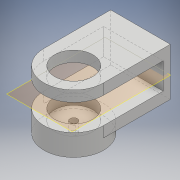
# Autodesk Inventor part: baseRotor1
Saved by Autodesk Inventor 2017 (Build 210142000, 142)
## iProperties
Created: 2017-08-06
Part Number: baseRotor1
Material: Generic
Document SubType Name: Sheet Metal
Designer: Bardo91
Density: 1 g/cm^3
Sheet Metal Rule: Default_mm
Appearance: Default
Author: Bardo91
Autodesk Inventor part; units mm, degrees
ref_plane "YZ Plane" through (0, 0, 0) normal (1, 0, 0) x (0, 1, 0)
ref_plane "XZ Plane" through (0, 0, 0) normal (0, 1, 0) x (-1, 0, 0)
ref_plane "XY Plane" through (0, 0, 0) normal (0, 0, 1) x (1, 0, 0)
sketch "Sketch1" plane through (0, 0, 0) normal (0, 0, 1) x (1, 0, 0)
  circle A0 centre (0, 0) radius 16
  circle A1 centre (0, 0) radius 25
  line L0 (-25, 0) -> (-25, 50)
  line L1 (-25, 50) -> (25, 50)
  line L2 (25, 50) -> (25, 0)
  dimension "d0" = 32
  dimension "d1" = 50
  dimension "d2" = 50
  dimension "d3" = 50
  constraints: 6 end point, 2 centre point, 2 coincident, 2 perpendicular, 2 point on circle, 1 vertical
  measures "d0" diameter of A0
  measures "d1" diameter of A1
  measures "d2" distance of L0.start L0.end
  measures "d3" distance of L0.end L1.end
extrude "Extrusion1" add sketch "Sketch1" along normal blind 9
ref_plane "Work Plane1" through (0, 0, -11) normal (0, 0, 1) x (1, 0, 0)
mirror "Mirror1" about plane through (0, 0, -11) normal (0, 0, 1) of "Extrusion1"
sketch "Sketch2" plane through (0, 0, -31) normal (0, 0, -1) x (-1, 0, 0)
  circle A0 centre (0, 0) radius 16 projected
  circle A1 centre (0, 0) radius 25
  dimension "d11" = 50
  constraints: 1 centre point, 1 coincident
  measures "d11" diameter of A1
extrude "Extrusion2" add sketch "Sketch2" along normal blind 9 contours A0 | A1
sketch "Sketch3" plane through (0, 0, -31) normal (0, 0, 1) x (1, 0, 0)
  circle A0 centre (0, 0) radius 3.1
  dimension "d14" = 6.2
  constraints: 1 centre point, 1 coincident
  measures "d14" diameter of A0
extrude "Extrusion3" cut sketch "Sketch3" against normal blind 1
sketch "Sketch4" plane through (0, 0, -32) normal (0, 0, 1) x (1, 0, 0)
  circle A0 centre (0, 0) radius 3.1
  line L0 (0, 0) -> (0, -1.5)
  line L1 (0, -1.5) -> (-2.7129, -1.5)
  line L2 (0, -1.5) -> (2.7129, -1.5)
  dimension "d17" = 6.2
  dimension "d18" = 1.5
  constraints: 6 end point, 2 horizontal, 2 point on circle, 1 centre point, 1 coincident, 1 vertical
  measures "d17" diameter of A0
  measures "d18" distance of L0.start L0.end
extrude "Extrusion4" cut sketch "Sketch4" against normal through all contours A0 L2 L1 picked at (-0.0193, 1.5513)
sketch "Sketch5" plane through (-25, 50, 0) normal (0, 1, 0) x (1, 0, 0)
  line L0 (0, 0) -> (0, -9) projected
  line L1 (0, 31) -> (50, 31) projected
  line L2 (0, -9) -> (50, -9)
  line L3 (50, -9) -> (50, 31)
  line L4 (50, 31) -> (0, 31)
  line L5 (0, 31) -> (0, -9)
  point P0 (25, 0)
  constraints: 8 end point, 2 parallel, 1 horizontal, 1 perpendicular
extrude "Extrusion5" add sketch "Sketch5" along normal blind 6
equation "\"BendRadius\" = Thickness"
equation "\"BendReliefWidth\" = Thickness"
equation "\"BendReliefDepth\" = 0.5 * Thickness"
equation "\"CornerReliefSize\" = 4 * Thickness"
equation "\"MinimumRemnant\" = 2 * Thickness"
equation "\"TransitionRadius\" = BendRadius"
equation "\"JacobiRadiusSize\" = BendRadius"
equation "\"GapSize\" = Thickness"
equation "\"Thickness\" = 0.5"
body "Solid1"
